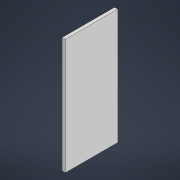
# Autodesk Inventor part: Sliding Plate
Saved by Autodesk Inventor 2022 (Build 260153000, 153)
## iProperties
Created: 2021-06-04
Part Number: Sliding Plate
Material: Generic
Document SubType Name: Modeling
Designer: saatvik123
Density: 1 g/cm^3
Appearance: Default
Author: saatvik123
## iProperties of the stored document Sliding Plate_3DPrint.ipt
Created: 2021-06-06
Part Number: Sliding Plate_3DPrint
Material: Generic
Document SubType Name: Modeling
Designer: sidsa
Density: 1 g/cm^3
Appearance: Default
Author: sidsa
Autodesk Inventor part; units mm, degrees
ref_plane "YZ Plane" through (0, 0, 0) normal (1, 0, 0) x (0, 1, 0)
ref_plane "XZ Plane" through (0, 0, 0) normal (0, 1, 0) x (-1, 0, 0)
ref_plane "XY Plane" through (0, 0, 0) normal (0, 0, 1) x (1, 0, 0)
sketch "Sketch1" plane through (0, 0, 0) normal (0, 0, 1) x (1, 0, 0)
  line L0 (17.78, -26.035) -> (20.32, -26.035) projected
  line L1 (20.32, -26.035) -> (20.32, -28.575) projected
  line L2 (22.86, -28.575) -> (20.32, -28.575) projected
  line L3 (22.86, -28.575) -> (22.86, -26.035) projected
  line L4 (22.86, -26.035) -> (25.4, -26.035) projected
  line L5 (25.4, 26.035) -> (25.4, -26.035) projected
  line L6 (25.4, 26.035) -> (22.86, 26.035) projected
  line L7 (22.86, 26.035) -> (22.86, 28.575) projected
  line L8 (20.32, 28.575) -> (22.86, 28.575) projected
  line L9 (20.32, 28.575) -> (20.32, 26.035) projected
  line L10 (20.32, 26.035) -> (17.78, 26.035) projected
  line L11 (-25.4, 28.575) -> (15.24, 28.575) projected
  line L12 (-25.4, -28.575) -> (-25.4, 28.575) projected
  line L13 (15.24, -28.575) -> (-25.4, -28.575) projected
  line L14 (20.32, -28.575) -> (22.86, -28.575)
  line L15 (22.86, -28.575) -> (22.86, 28.575)
  line L16 (22.86, 28.575) -> (20.32, 28.575)
  line L17 (20.32, 28.575) -> (20.32, -28.575)
  line L18 (20.828, -28.067) -> (22.352, -28.067)
  line L19 (22.352, -28.067) -> (22.352, 28.067)
  line L20 (22.352, 28.067) -> (20.828, 28.067)
  line L21 (20.828, 28.067) -> (20.828, -28.067)
  line L22 (17.78, -26.035) -> (15.24, -28.575) projected
  line L23 (15.24, 28.575) -> (17.78, 26.035) projected
  point P0 (0, 0)
  dimension "d0" = 0.508
  constraints: 16 end point, 4 parallel, 2 perpendicular, 1 horizontal, 3 other
  measures "d0" distance between parallel lines of L17 L21
extrude "Extrusion1" add sketch "Sketch1" along normal blind 25.4 contours L21 L20 L19 L18
body "Solid1"
